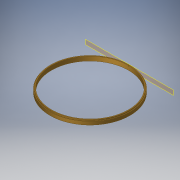
# Autodesk Inventor part: 4K sheild rim3
Saved by Autodesk Inventor 2018 (Build 220112000, 112)
## iProperties
Created: 2019-03-11
Part Number: 4K sheild rim3
Material: Brass, Soft Yellow
Document SubType Name: Modeling
Designer: Admin
Density: 8.47 g/cm^3
Appearance: Brass - Satin
Author: Admin
Autodesk Inventor part; units mm, degrees
ref_plane "YZ Plane" through (0, 0, 0) normal (1, 0, 0) x (0, 1, 0)
ref_plane "XZ Plane" through (0, 0, 0) normal (0, 1, 0) x (-1, 0, 0)
sketch "Sketch1" plane through (0, 0, 0) normal (0, 1, 0) x (-1, 0, 0)
  circle A0 centre (0, 0) radius 98.425
  circle A1 centre (0, 0) radius 102.489
  dimension "d0" = 196.85
  dimension "d1" = 4.064
  constraints: 2 centre point, 2 coincident
  measures "d0" diameter of A0
  measures "d1" radial gap between concentric circles of A1 A0
extrude "Extrusion1" add sketch "Sketch1" along normal blind 8.255
sketch "Sketch2" plane through (0, 8.255, 0) normal (0, 1, 0) x (1, 0, 0)
  circle A0 centre (0, 0) radius 98.425
  circle A1 centre (0, 0) radius 98.425 projected
  circle A2 centre (0, 0) radius 100.838
  dimension "d4" = 2.413
  constraints: 2 centre point, 2 coincident, 1 concentric
  measures "d4" radial gap between concentric circles of A2 A0
extrude "Extrusion2" add sketch "Sketch2" along normal blind 2.413
ref_plane "Work Plane1" through (0, 8.255, -100.838) normal (0, 0, 1) x (1, 0, 0)
sketch "Sketch3" plane through (0, 8.255, -100.838) normal (0, 0, 1) x (1, 0, 0)
  line L0 (102.489, 0) -> (-102.489, 0) construction
  line L1 (0, 0) -> (0, 1.27) construction
  point P0 (0, -8.255)
  dimension "d7" = 1.27
  constraints: 2 end point, 1 coincident, 1 midpoint, 1 vertical
  measures "d7" distance of L1.start L1.end
hole "Hole1" at (0, 9.525, -100.838) direction (0, 0, 1) diameter 1.5748 depth 6.2992 tip angle 118
pattern_circular "Circular Pattern1" count 6 over 360 about axis through (0, 0, 0) along (0, 1, 0) of "Hole1"
body "Solid1"
